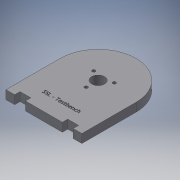
# Autodesk Inventor part: Support_motor_front
Saved by Autodesk Inventor 2017 (Build 210142000, 142)
## iProperties
Part Number: Support_motor_front
Material: Générique
Document SubType Name: Modeling
Designer: Darren
Density: 1 g/cm^3
Appearance: Par défaut
Author: Darren
Autodesk Inventor part; units mm, degrees
ref_plane "YZ Plane" through (0, 0, 0) normal (1, 0, 0) x (0, 1, 0)
ref_plane "XZ Plane" through (0, 0, 0) normal (0, 1, 0) x (-1, 0, 0)
ref_plane "XY Plane" through (0, 0, 0) normal (0, 0, 1) x (1, 0, 0)
sketch "Esquisse1" plane through (0, 0, 0) normal (0, 0, 1) x (1, 0, 0)
  line L0 (-49, 0) -> (49, 0) construction
  line L1 (0, -67) -> (0, 52) construction
  circle A0 centre (0, 0) radius 6
  circle A1 centre (0, 0) radius 11 construction
  line L2 (0, 0) -> (-9.5263, 5.5) construction
  circle A2 centre (-9.5263, 5.5) radius 1.5
  circle A3 centre (0, -11) radius 1.5
  circle A4 centre (9.5263, 5.5) radius 1.5
  circle A5 centre (0, 0) radius 30 construction
  line L3 (0, 0) -> (35, 0) construction
  line L4 (0, 0) -> (35, 0) construction
  line L5 (0, 0) -> (-35, 0) construction
  line L6 (-35, 0) -> (35, 0) construction
  line L7 (35, 0) -> (35, -50)
  line L8 (-35, -50) -> (-35, 0)
  line L9 (-17, -50) -> (-17, -45)
  line L10 (-17, -45) -> (-27, -45)
  line L11 (-27, -45) -> (-27, -50)
  line L12 (27, -50) -> (27, -45)
  line L13 (27, -45) -> (17, -45)
  line L14 (17, -45) -> (17, -50)
  line L15 (-27, -50) -> (-35, -50)
  line L16 (35, -50) -> (27, -50)
  line L17 (17, -50) -> (-17, -50)
  arc A6 (35, 0) -> (-35, 0) centre (0, 0) ccw
  line L18 (0, 0) -> (9.5263, 5.5) construction
  line L19 (0, 0) -> (0, -11) construction
  dimension "d0" = 12
  dimension "d1" = 22
  dimension "d4" = 11
  dimension "d5" = 30
  dimension "d6" = 3
  dimension "d9" = 360
  dimension "d11" = 60
  dimension "d15" = 0
  dimension "d16" = 180
  dimension "d19" = 10
  dimension "d21" = 10
  dimension "d23" = 8
  dimension "d24" = 8
  dimension "d25" = 50
  dimension "d26" = 70
  dimension "d28" = 5
  dimension "d29" = 5
  dimension "d30" = 5
  dimension "d31" = 5
  constraints: 36 end point, 8 coincident, 7 centre point, 6 parallel, 2 horizontal, 2 point on circle, 1 collinear, 1 perpendicular, 10 other
  measures "d0" diameter of A0
  measures "d1" diameter of A1
  measures "d4" distance of L2.start L2.end
  measures "d5" angle of L0 L2
  measures "d6" diameter of A2
  measures "d11" diameter of A5
  measures "d15" distance between parallel lines of L3 L4
  measures "d16" angle of L5 L3
  measures "d19" distance of L10.end L9.end
  measures "d21" distance of L13.end L12.end
  measures "d23" distance between parallel lines of L7 L12
  measures "d24" distance between parallel lines of L8 L11
  measures "d25" distance between parallel lines of L16 L6
  measures "d26" distance between parallel lines of L8 L7
  measures "d28" distance between parallel lines of L10 L17
  measures "d29" distance between parallel lines of L10 L15
  measures "d30" distance between parallel lines of L16 L13
  measures "d31" distance between parallel lines of L13 L17
extrude "Extrusion1" add sketch "Esquisse1" along normal blind 8
sketch "Esquisse2" plane through (0, 0, 8) normal (0, 0, 1) x (1, 0, 0)
  circle A0 centre (0, 0) radius 6 projected
  circle A1 centre (9.5263, 5.5) radius 1.5 projected
  circle A2 centre (0, -11) radius 1.5 projected
  circle A3 centre (-9.5263, 5.5) radius 1.5 projected
  line L0 (35, -50) -> (35, 0) projected
  arc A4 (35, 0) -> (-35, 0) centre (0, 0) ccw projected
  line L1 (-35, 0) -> (-35, -50) projected
  line L2 (-35, -50) -> (-27, -50) projected
  line L3 (-27, -50) -> (-27, -45) projected
  line L4 (-27, -45) -> (-17, -45) projected
  line L5 (-17, -45) -> (-17, -50) projected
  line L6 (-17, -50) -> (17, -50) projected
  line L7 (17, -50) -> (17, -45) projected
  line L8 (17, -45) -> (27, -45) projected
  line L9 (27, -45) -> (27, -50) projected
  line L10 (27, -50) -> (35, -50) projected
  line L11 (-28.0795, -27.4274) -> (28.6834, -27.4274) construction
  line L12 (28.6834, -27.4274) -> (28.6834, -39.9575) construction
  line L13 (28.6834, -39.9575) -> (-28.0795, -39.9575) construction
  line L14 (-28.0795, -39.9575) -> (-28.0795, -27.4274) construction
  line L15 (-16.5276, -35.2865) -> (-16.3552, -34.8514)
  spline S0 degree 2 poles (-16.3552, -34.8514) (-16.2239, -34.9472) (-15.8298, -35.0785) (-15.6738, -35.0785) knots 0 0 0 1 2 2 2
  spline S1 degree 2 poles (-15.6738, -35.0785) (-15.3974, -35.0785) (-15.0636, -34.7775) (-15.0636, -34.5422) knots 0 0 0 1 2 2 2
  spline S2 degree 2 poles (-15.0636, -34.5422) (-15.0636, -34.3698) (-15.2497, -34.0687) (-15.6246, -33.8936) knots 0 0 0 1 2 2 2
  line L16 (-15.6246, -33.8936) -> (-15.901, -33.7622)
  spline S3 degree 2 poles (-15.901, -33.7622) (-16.2567, -33.5981) (-16.5358, -33.1465) (-16.5358, -32.8264) knots 0 0 0 1 2 2 2
  spline S4 degree 2 poles (-16.5358, -32.8264) (-16.5358, -32.4405) (-15.9885, -31.9315) (-15.5616, -31.9315) knots 0 0 0 1 2 2 2
  spline S5 degree 2 poles (-15.5616, -31.9315) (-14.9897, -31.9315) (-14.7653, -32.1176) knots 0 0 0 1 1 1
  line L17 (-14.7653, -32.1176) -> (-14.9049, -32.5281)
  spline S6 degree 2 poles (-14.9049, -32.5281) (-14.9979, -32.4597) (-15.3838, -32.3311) (-15.5507, -32.3311) knots 0 0 0 1 2 2 2
  spline S7 degree 2 poles (-15.5507, -32.3311) (-15.7888, -32.3311) (-16.0652, -32.6047) (-16.0652, -32.8182) knots 0 0 0 1 2 2 2
  spline S8 degree 2 poles (-16.0652, -32.8182) (-16.0652, -32.9522) (-15.9666, -33.1684) (-15.7888, -33.3162) (-15.5151, -33.4475) knots 0 0 0 1 2 3 3 3
  line L18 (-15.5151, -33.4475) -> (-15.2333, -33.5816)
  spline S9 degree 2 poles (-15.2333, -33.5816) (-14.8802, -33.7486) (-14.5956, -34.2138) (-14.5956, -34.5723) knots 0 0 0 1 2 2 2
  spline S10 degree 2 poles (-14.5956, -34.5723) (-14.5956, -34.9608) (-15.2196, -35.5027) (-15.7422, -35.5027) knots 0 0 0 1 2 2 2
  spline S11 degree 2 poles (-15.7422, -35.5027) (-16.202, -35.5027) (-16.5276, -35.2865) knots 0 0 0 1 1 1
  line L19 (-14.2071, -35.2865) -> (-14.0347, -34.8514)
  spline S12 degree 2 poles (-14.0347, -34.8514) (-13.9033, -34.9472) (-13.5093, -35.0785) (-13.3533, -35.0785) knots 0 0 0 1 2 2 2
  spline S13 degree 2 poles (-13.3533, -35.0785) (-13.0769, -35.0785) (-12.743, -34.7775) (-12.743, -34.5422) knots 0 0 0 1 2 2 2
  spline S14 degree 2 poles (-12.743, -34.5422) (-12.743, -34.3698) (-12.9291, -34.0687) (-13.304, -33.8936) knots 0 0 0 1 2 2 2
  line L20 (-13.304, -33.8936) -> (-13.5804, -33.7622)
  spline S15 degree 2 poles (-13.5804, -33.7622) (-13.9361, -33.5981) (-14.2153, -33.1465) (-14.2153, -32.8264) knots 0 0 0 1 2 2 2
  spline S16 degree 2 poles (-14.2153, -32.8264) (-14.2153, -32.4405) (-13.668, -31.9315) (-13.2411, -31.9315) knots 0 0 0 1 2 2 2
  spline S17 degree 2 poles (-13.2411, -31.9315) (-12.6691, -31.9315) (-12.4447, -32.1176) knots 0 0 0 1 1 1
  line L21 (-12.4447, -32.1176) -> (-12.5843, -32.5281)
  spline S18 degree 2 poles (-12.5843, -32.5281) (-12.6774, -32.4597) (-13.0632, -32.3311) (-13.2301, -32.3311) knots 0 0 0 1 2 2 2
  spline S19 degree 2 poles (-13.2301, -32.3311) (-13.4682, -32.3311) (-13.7446, -32.6047) (-13.7446, -32.8182) knots 0 0 0 1 2 2 2
  spline S20 degree 2 poles (-13.7446, -32.8182) (-13.7446, -32.9522) (-13.6461, -33.1684) (-13.4682, -33.3162) (-13.1946, -33.4475) knots 0 0 0 1 2 3 3 3
  line L22 (-13.1946, -33.4475) -> (-12.9127, -33.5816)
  spline S21 degree 2 poles (-12.9127, -33.5816) (-12.5597, -33.7486) (-12.2751, -34.2138) (-12.2751, -34.5723) knots 0 0 0 1 2 2 2
  spline S22 degree 2 poles (-12.2751, -34.5723) (-12.2751, -34.9608) (-12.899, -35.5027) (-13.4217, -35.5027) knots 0 0 0 1 2 2 2
  spline S23 degree 2 poles (-13.4217, -35.5027) (-13.8814, -35.5027) (-14.2071, -35.2865) knots 0 0 0 1 1 1
  line L23 (-11.7305, -35.4425) -> (-11.7305, -31.989)
  line L24 (-11.7305, -31.989) -> (-11.2598, -31.989)
  line L25 (-11.2598, -31.989) -> (-11.2598, -35.0183)
  line L26 (-11.2598, -35.0183) -> (-9.7, -35.0183)
  line L27 (-9.7, -35.0183) -> (-9.7, -35.4425)
  line L28 (-9.7, -35.4425) -> (-11.7305, -35.4425)
  line L29 (-7.8118, -34.2493) -> (-7.8118, -33.8361)
  line L30 (-7.8118, -33.8361) -> (-6.8021, -33.8361)
  line L31 (-6.8021, -33.8361) -> (-6.8021, -34.2493)
  line L32 (-6.8021, -34.2493) -> (-7.8118, -34.2493)
  line L33 (-3.3486, -32.4131) -> (-3.3486, -35.4425)
  line L34 (-3.3486, -35.4425) -> (-3.8193, -35.4425)
  line L35 (-3.8193, -35.4425) -> (-3.8193, -32.4131)
  line L36 (-3.8193, -32.4131) -> (-4.9166, -32.4131)
  line L37 (-4.9166, -32.4131) -> (-4.9166, -31.989)
  line L38 (-4.9166, -31.989) -> (-2.202, -31.989)
  line L39 (-2.202, -31.989) -> (-2.202, -32.4131)
  line L40 (-2.202, -32.4131) -> (-3.3486, -32.4131)
  line L41 (0.2855, -34.222) -> (-1.5343, -34.222)
  spline S24 degree 2 poles (-1.5343, -34.222) (-1.5343, -34.6653) (-1.2907, -34.9034) knots 0 0 0 1 1 1
  spline S25 degree 2 poles (-1.2907, -34.9034) (-1.0773, -35.1113) (-0.7379, -35.1113) knots 0 0 0 1 1 1
  spline S26 degree 2 poles (-0.7379, -35.1113) (-0.3548, -35.1113) (-0.0976, -34.887) knots 0 0 0 1 1 1
  line L42 (-0.0976, -34.887) -> (0.0912, -35.2099)
  spline S27 degree 2 poles (0.0912, -35.2099) (-0.0128, -35.3139) (-0.2262, -35.3905) knots 0 0 0 1 1 1
  spline S28 degree 2 poles (-0.2262, -35.3905) (-0.4971, -35.489) (-0.8255, -35.489) knots 0 0 0 1 1 1
  spline S29 degree 2 poles (-0.8255, -35.489) (-1.3017, -35.489) (-1.6355, -35.1661) knots 0 0 0 1 1 1
  spline S30 degree 2 poles (-1.6355, -35.1661) (-2.005, -34.8103) (-2.005, -34.2083) knots 0 0 0 1 1 1
  spline S31 degree 2 poles (-2.005, -34.2083) (-2.005, -33.5844) (-1.6246, -33.2067) knots 0 0 0 1 1 1
  spline S32 degree 2 poles (-1.6246, -33.2067) (-1.2852, -32.8701) (-0.8228, -32.8701) knots 0 0 0 1 1 1
  spline S33 degree 2 poles (-0.8228, -32.8701) (-0.2809, -32.8701) (0.0228, -33.1739) knots 0 0 0 1 1 1
  spline S34 degree 2 poles (0.0228, -33.1739) (0.3211, -33.4667) (0.3211, -33.9483) knots 0 0 0 1 1 1
  spline S35 degree 2 poles (0.3211, -33.9483) (0.3211, -34.0961) (0.2855, -34.222) knots 0 0 0 1 1 1
  spline S36 degree 2 poles (-0.8009, -33.2478) (-1.0992, -33.2478) (-1.3017, -33.4393) knots 0 0 0 1 1 1
  spline S37 degree 2 poles (-1.3017, -33.4393) (-1.496, -33.6227) (-1.5206, -33.8963) knots 0 0 0 1 1 1
  line L43 (-1.5206, -33.8963) -> (-0.125, -33.8963)
  spline S38 degree 2 poles (-0.125, -33.8963) (-0.125, -33.6254) (-0.2946, -33.4448) knots 0 0 0 1 1 1
  spline S39 degree 2 poles (-0.2946, -33.4448) (-0.4807, -33.2478) (-0.8009, -33.2478) knots 0 0 0 1 1 1
  line L44 (0.6276, -35.292) -> (0.7863, -34.8678)
  spline S40 degree 2 poles (0.7863, -34.8678) (1.1612, -35.1113) (1.3883, -35.1113) knots 0 0 0 1 1 1
  spline S41 degree 2 poles (1.3883, -35.1113) (1.8043, -35.1113) (1.8043, -34.7638) knots 0 0 0 1 1 1
  spline S42 degree 2 poles (1.8043, -34.7638) (1.8043, -34.5121) (1.4047, -34.3342) knots 0 0 0 1 1 1
  spline S43 degree 2 poles (1.4047, -34.3342) (1.0955, -34.1919) (0.8793, -34.0468) (0.7206, -33.8608) (0.644, -33.6501) (0.644, -33.5296) knots 0 0 0 1 2 3 4 4 4
  spline S44 degree 2 poles (0.644, -33.5296) (0.644, -33.2177) (1.0955, -32.8701) (1.4622, -32.8701) knots 0 0 0 1 2 2 2
  spline S45 degree 2 poles (1.4622, -32.8701) (1.7386, -32.8701) (2.1573, -33.0453) knots 0 0 0 1 1 1
  line L45 (2.1573, -33.0453) -> (2.0287, -33.4585)
  spline S46 degree 2 poles (2.0287, -33.4585) (1.7632, -33.2478) (1.495, -33.2478) knots 0 0 0 1 1 1
  spline S47 degree 2 poles (1.495, -33.2478) (1.3336, -33.2478) (1.1147, -33.3983) (1.1147, -33.5132) knots 0 0 0 1 2 2 2
  spline S48 degree 2 poles (1.1147, -33.5132) (1.1147, -33.7568) (1.3911, -33.8827) knots 0 0 0 1 1 1
  line L46 (1.3911, -33.8827) -> (1.7112, -34.0277)
  spline S49 degree 2 poles (1.7112, -34.0277) (2.0068, -34.1618) (2.275, -34.5066) (2.275, -34.7665) knots 0 0 0 1 2 2 2
  spline S50 degree 2 poles (2.275, -34.7665) (2.275, -35.1059) (1.7988, -35.489) (1.3774, -35.489) knots 0 0 0 1 2 2 2
  spline S51 degree 2 poles (1.3774, -35.489) (0.9778, -35.489) (0.6276, -35.292) knots 0 0 0 1 1 1
  line L47 (2.9071, -33.2724) -> (2.6143, -33.2724)
  line L48 (2.6143, -33.2724) -> (2.6143, -32.9194)
  line L49 (2.6143, -32.9194) -> (2.9071, -32.9194)
  line L50 (2.9071, -32.9194) -> (2.9071, -32.3913)
  line L51 (2.9071, -32.3913) -> (3.3559, -32.2189)
  line L52 (3.3559, -32.2189) -> (3.3559, -32.9194)
  line L53 (3.3559, -32.9194) -> (4.0482, -32.9194)
  line L54 (4.0482, -32.9194) -> (4.0482, -33.2724)
  line L55 (4.0482, -33.2724) -> (3.3559, -33.2724)
  line L56 (3.3559, -33.2724) -> (3.3559, -34.5257)
  spline S52 degree 2 poles (3.3559, -34.5257) (3.3559, -34.8432) (3.5693, -35.1113) (3.8074, -35.1113) knots 0 0 0 1 2 2 2
  spline S53 degree 2 poles (3.8074, -35.1113) (3.9798, -35.1113) (4.1631, -35.0238) knots 0 0 0 1 1 1
  line L57 (4.1631, -35.0238) -> (4.2288, -35.4178)
  spline S54 degree 2 poles (4.2288, -35.4178) (3.9497, -35.489) (3.6186, -35.489) knots 0 0 0 1 1 1
  spline S55 degree 2 poles (3.6186, -35.489) (3.3203, -35.489) (2.9071, -35.0429) (2.9071, -34.7036) knots 0 0 0 1 2 2 2
  line L58 (2.9071, -34.7036) -> (2.9071, -33.2724)
  line L59 (5.0416, -35.2591) -> (4.8829, -35.489)
  line L60 (4.8829, -35.489) -> (4.6585, -35.489)
  line L61 (4.6585, -35.489) -> (4.6585, -31.8823)
  line L62 (4.6585, -31.8823) -> (5.1072, -31.8823)
  line L63 (5.1072, -31.8823) -> (5.1072, -33.1027)
  spline S56 degree 2 poles (5.1072, -33.1027) (5.1702, -33.0152) (5.5232, -32.8701) (5.6929, -32.8701) knots 0 0 0 1 2 2 2
  spline S57 degree 2 poles (5.6929, -32.8701) (6.2101, -32.8701) (6.8531, -33.5871) (6.8531, -34.1344) knots 0 0 0 1 2 2 2
  spline S58 degree 2 poles (6.8531, -34.1344) (6.8531, -34.7665) (6.2073, -35.489) (5.6545, -35.489) knots 0 0 0 1 2 2 2
  spline S59 degree 2 poles (5.6545, -35.489) (5.4767, -35.489) (5.1291, -35.3549) (5.0416, -35.2591) knots 0 0 0 1 2 2 2
  line L64 (5.1072, -33.4448) -> (5.1072, -34.9006)
  spline S60 degree 2 poles (5.1072, -34.9006) (5.1072, -34.9389) (5.4411, -35.1113) (5.5287, -35.1113) knots 0 0 0 1 2 2 2
  spline S61 degree 2 poles (5.5287, -35.1113) (5.9857, -35.1113) (6.3825, -34.6735) (6.3825, -34.1563) knots 0 0 0 1 2 2 2
  spline S62 degree 2 poles (6.3825, -34.1563) (6.3825, -33.7294) (5.92, -33.2478) (5.5287, -33.2478) knots 0 0 0 1 2 2 2
  spline S63 degree 2 poles (5.5287, -33.2478) (5.4466, -33.2478) (5.151, -33.3901) (5.1072, -33.4448) knots 0 0 0 1 2 2 2
  line L65 (9.4747, -34.222) -> (7.6549, -34.222)
  spline S64 degree 2 poles (7.6549, -34.222) (7.6549, -34.6653) (7.8985, -34.9034) knots 0 0 0 1 1 1
  spline S65 degree 2 poles (7.8985, -34.9034) (8.1119, -35.1113) (8.4513, -35.1113) knots 0 0 0 1 1 1
  spline S66 degree 2 poles (8.4513, -35.1113) (8.8344, -35.1113) (9.0916, -34.887) knots 0 0 0 1 1 1
  line L66 (9.0916, -34.887) -> (9.2804, -35.2099)
  spline S67 degree 2 poles (9.2804, -35.2099) (9.1764, -35.3139) (8.963, -35.3905) knots 0 0 0 1 1 1
  spline S68 degree 2 poles (8.963, -35.3905) (8.6921, -35.489) (8.3637, -35.489) knots 0 0 0 1 1 1
  spline S69 degree 2 poles (8.3637, -35.489) (7.8875, -35.489) (7.5537, -35.1661) knots 0 0 0 1 1 1
  spline S70 degree 2 poles (7.5537, -35.1661) (7.1843, -34.8103) (7.1843, -34.2083) knots 0 0 0 1 1 1
  spline S71 degree 2 poles (7.1843, -34.2083) (7.1843, -33.5844) (7.5646, -33.2067) knots 0 0 0 1 1 1
  spline S72 degree 2 poles (7.5646, -33.2067) (7.904, -32.8701) (8.3664, -32.8701) knots 0 0 0 1 1 1
  spline S73 degree 2 poles (8.3664, -32.8701) (8.9083, -32.8701) (9.212, -33.1739) knots 0 0 0 1 1 1
  spline S74 degree 2 poles (9.212, -33.1739) (9.5103, -33.4667) (9.5103, -33.9483) knots 0 0 0 1 1 1
  spline S75 degree 2 poles (9.5103, -33.9483) (9.5103, -34.0961) (9.4747, -34.222) knots 0 0 0 1 1 1
  spline S76 degree 2 poles (8.3883, -33.2478) (8.09, -33.2478) (7.8875, -33.4393) knots 0 0 0 1 1 1
  spline S77 degree 2 poles (7.8875, -33.4393) (7.6933, -33.6227) (7.6686, -33.8963) knots 0 0 0 1 1 1
  line L67 (7.6686, -33.8963) -> (9.0642, -33.8963)
  spline S78 degree 2 poles (9.0642, -33.8963) (9.0642, -33.6254) (8.8946, -33.4448) knots 0 0 0 1 1 1
  spline S79 degree 2 poles (8.8946, -33.4448) (8.7085, -33.2478) (8.3883, -33.2478) knots 0 0 0 1 1 1
  line L68 (11.5353, -35.4425) -> (11.5353, -33.973)
  spline S80 degree 2 poles (11.5353, -33.973) (11.5353, -33.5707) (11.2918, -33.2478) (11.0072, -33.2478) knots 0 0 0 1 2 2 2
  spline S81 degree 2 poles (11.0072, -33.2478) (10.8539, -33.2478) (10.5201, -33.4311) (10.4298, -33.5652) knots 0 0 0 1 2 2 2
  line L69 (10.4298, -33.5652) -> (10.4298, -35.4425)
  line L70 (10.4298, -35.4425) -> (9.981, -35.4425)
  line L71 (9.981, -35.4425) -> (9.981, -32.9194)
  line L72 (9.981, -32.9194) -> (10.2875, -32.9194)
  line L73 (10.2875, -32.9194) -> (10.4298, -33.245)
  spline S82 degree 2 poles (10.4298, -33.245) (10.6514, -32.8701) (11.1549, -32.8701) knots 0 0 0 1 1 1
  spline S83 degree 2 poles (11.1549, -32.8701) (11.9841, -32.8701) (11.9841, -33.8799) knots 0 0 0 1 1 1
  line L74 (11.9841, -33.8799) -> (11.9841, -35.4425)
  line L75 (11.9841, -35.4425) -> (11.5353, -35.4425)
  line L76 (14.5373, -33.1219) -> (14.3129, -33.4366)
  spline S84 degree 2 poles (14.3129, -33.4366) (14.2445, -33.3682) (13.8942, -33.2478) (13.7273, -33.2478) knots 0 0 0 1 2 2 2
  spline S85 degree 2 poles (13.7273, -33.2478) (13.3578, -33.2478) (12.9255, -33.7595) (12.9255, -34.2056) knots 0 0 0 1 2 2 2
  spline S86 degree 2 poles (12.9255, -34.2056) (12.9255, -34.6461) (13.3633, -35.1113) (13.7519, -35.1113) knots 0 0 0 1 2 2 2
  spline S87 degree 2 poles (13.7519, -35.1113) (14.0529, -35.1113) (14.3594, -34.8787) knots 0 0 0 1 1 1
  line L77 (14.3594, -34.8787) -> (14.5373, -35.2564)
  spline S88 degree 2 poles (14.5373, -35.2564) (14.176, -35.489) (13.6452, -35.489) knots 0 0 0 1 1 1
  spline S89 degree 2 poles (13.6452, -35.489) (13.128, -35.489) (12.4548, -34.7967) (12.4548, -34.2056) knots 0 0 0 1 2 2 2
  spline S90 degree 2 poles (12.4548, -34.2056) (12.4548, -33.6008) (13.1581, -32.8701) (13.771, -32.8701) knots 0 0 0 1 2 2 2
  spline S91 degree 2 poles (13.771, -32.8701) (13.9681, -32.8701) (14.4278, -33.0343) (14.5373, -33.1219) knots 0 0 0 1 2 2 2
  line L78 (16.5623, -35.4425) -> (16.5623, -33.8553)
  spline S92 degree 2 poles (16.5623, -33.8553) (16.5623, -33.5734) (16.2859, -33.2478) (16.0341, -33.2478) knots 0 0 0 1 2 2 2
  spline S93 degree 2 poles (16.0341, -33.2478) (15.87, -33.2478) (15.5443, -33.4393) (15.4567, -33.5652) knots 0 0 0 1 2 2 2
  line L79 (15.4567, -33.5652) -> (15.4567, -35.4425)
  line L80 (15.4567, -35.4425) -> (15.0079, -35.4425)
  line L81 (15.0079, -35.4425) -> (15.0079, -31.8823)
  line L82 (15.0079, -31.8823) -> (15.4567, -31.8823)
  line L83 (15.4567, -31.8823) -> (15.4567, -33.1958)
  spline S94 degree 2 poles (15.4567, -33.1958) (15.547, -33.0562) (15.9438, -32.8701) (16.1573, -32.8701) knots 0 0 0 1 2 2 2
  spline S95 degree 2 poles (16.1573, -32.8701) (16.5568, -32.8701) (17.0111, -33.3983) (17.0111, -33.8553) knots 0 0 0 1 2 2 2
  line L84 (17.0111, -33.8553) -> (17.0111, -35.4425)
  line L85 (17.0111, -35.4425) -> (16.5623, -35.4425)
  constraints: 2 other
emboss "Gravure1" sketch "Esquisse2" operation cut depth 1 direction (0, 0, -1) contours L15 S0 S1 S2 L16 S3 S4 S5 L17 S6 S7 S8 L18 S9 S10 S11 | L19 S12 S13 S14 L20 S15 S16 S17 L21 S18 S19 S20 L22 S21 S22 S23 | L23 L24 L25 L26 L27 L28 | L29 L30 L31 L32 | L33 L34 L35 L36 L37 L38 L39 L40 | L41 S24 S25 S26 L42 S27 S28 S29 S30 S31 S32 S33 S34 S35 | L44 S40 S41 S42 S43 S44 S45 L45 S46 S47 S48 L46 S49 S50 S51 | L47 L48 L49 L50 L51 L52 L53 L54 L55 L56 S52 S53 L57 S54 S55 L58 | L59 L60 L61 L62 L63 S56 S57 S58 S59 | L65 S64 S65 S66 L66 S67 S68 S69 S70 S71 S72 S73 S74 S75 | L68 S80 S81 L69 L70 L71 L72 L73 S82 S83 L74 L75 | L76 S84 S85 S86 S87 L77 S88 S89 S90 S91 | L78 S92 S93 L79 L80 L81 L82 L83 S94 S95 L84 L85
